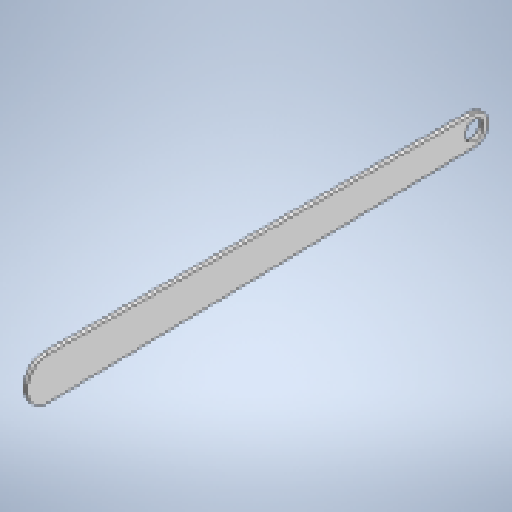
# Autodesk Inventor part: 4BarArm2.0
Saved by Autodesk Inventor 2023 (Build 270158000, 158)
## iProperties
Created: 2022-10-13
Part Number: 4BarArm2.0
Material: Generic
Document SubType Name: Modeling
Designer: deli
Density: 1 g/cm^3
Appearance: Default
Author: deli
Autodesk Inventor part; units mm, degrees
ref_plane "YZ Plane" through (0, 0, 0) normal (1, 0, 0) x (0, 1, 0)
ref_plane "XZ Plane" through (0, 0, 0) normal (0, 1, 0) x (-1, 0, 0)
ref_plane "XY Plane" through (0, 0, 0) normal (0, 0, 1) x (1, 0, 0)
sketch "Sketch1" plane through (0, 0, 0) normal (1, 0, 0) x (0, 1, 0)
  arc A0 (28.5717, 100.1291) -> (-3.4242, 100.0062) centre (12.5728, 100.3154) ccw
  circle A1 centre (13.8134, -222.6823) radius 7
  arc A2 (2.8155, -222.8948) -> (24.8127, -222.8103) centre (13.8134, -222.6823) ccw
  line L0 (28.5717, 100.1291) -> (24.8127, -222.8103)
  line L1 (-3.4242, 100.0062) -> (2.8155, -222.8948)
  point P0 (0, 0)
  dimension "d0" = 32
  dimension "d1" = 14
  dimension "d2" = 4
  dimension "d3" = 323
  constraints: 4 end point, 4 point on circle, 4 tangent, 3 centre point, 1 coincident
  measures "d0" diameter of A0
  measures "d1" diameter of A1
  measures "d2" radial gap between concentric circles of A2 A1
  measures "d3" distance of A1.centre A0.centre
extrude "Extrusion1" add sketch "Sketch1" along normal blind 3.175
body "Solid1"
